Autodesk Fusion 360 part; units mm, degrees
(part 2 of 2)
sketch "Sketch1" plane through (0, 0, 0) normal (0, 0, 1) x (1, 0, 0)
  circle A0 centre (0, 0) radius 2
  circle A1 centre (0, 0) radius 7.85
  dimension "d1" = 4
  dimension "d2" = 15.7
  constraint coincident A0.centre A1.centre
  measures "d1" diameter of A0
  measures "d2" diameter of A1
extrude "Extrude1" add sketch "Sketch1" along normal blind 1 contours A0 | A1
extrude "Extrude2" add sketch "Sketch1" along normal blind 3 contours A0
sketch "Sketch2" plane through (0, 0, 3) normal (0, 0, 1) x (-1, 0, 0)
  circle A0 centre (0, 0) radius 2
  circle A1 centre (0, 0) radius 0.75
  dimension "d7" = 1.5
  constraint concentric A0 A1
  measures "d7" diameter of A1
extrude "Extrude3" cut sketch "Sketch2" against normal blind 7 contours A1
sketch "Sketch3" plane through (0, 0, 3) normal (0, 0, 1) x (-1, 0, 0)
  circle A0 centre (0, 0) radius 0.75
  circle A1 centre (0, 0) radius 2
  circle A2 centre (0, 0) radius 2
  line L0 (0.35, -1.9691) -> (0, -1.3629)
  line L1 (0, -1.3629) -> (-0.35, -1.9691)
  dimension "d10" = 0.7
  dimension "d11" = 0.7
  constraint coincident A0.centre A1.centre
  constraint coincident A1 L0.start
  constraint coincident A2 L1.end
  constraint equal L0 L1
  constraint vertical A0.centre L0.end
  constraint equal A1 A2
  measures "d10" distance of L0.start L0.end
  measures "d11" horizontal distance of L0.start L1.end
extrude "Extrude4" cut sketch "Sketch3" against normal blind 2 contours A1 A2 L0 L1 picked at (0, -1.7853)
pattern_circular "C-Pattern1" count 12 over 360 about axis through (0, 0, 3) along (0, 0, -1) of "Extrude4"
sketch "Sketch4" plane through (0, 0, 1) normal (0, 0, 1) x (-1, 0, 0)
  line L0 (-0.6815, -1.8803) -> (-0.6815, -1.1803)
  line L1 (-0.6815, -1.1803) -> (-1.2877, -1.5303)
  line L2 (-1.5303, -1.2877) -> (-1.1803, -0.6815)
  line L3 (-1.1803, -0.6815) -> (-1.8803, -0.6815)
  line L4 (-1.9691, -0.35) -> (-1.3629, 0)
  line L5 (-1.3629, 0) -> (-1.9691, 0.35)
  line L6 (-1.8803, 0.6815) -> (-1.1803, 0.6815)
  line L7 (-1.1803, 0.6815) -> (-1.5303, 1.2877)
  line L8 (-1.2877, 1.5303) -> (-0.6815, 1.1803)
  line L9 (-0.6815, 1.1803) -> (-0.6815, 1.8803)
  line L10 (-0.35, 1.9691) -> (0, 1.3629)
  line L11 (0, 1.3629) -> (0.35, 1.9691)
  line L12 (0.6815, 1.8803) -> (0.6815, 1.1803)
  line L13 (0.6815, 1.1803) -> (1.2877, 1.5303)
  line L14 (1.5303, 1.2877) -> (1.1803, 0.6815)
  line L15 (1.1803, 0.6815) -> (1.8803, 0.6815)
  line L16 (1.9691, 0.35) -> (1.3629, 0)
  line L17 (1.3629, 0) -> (1.9691, -0.35)
  line L18 (1.8803, -0.6815) -> (1.1803, -0.6815)
  line L19 (1.1803, -0.6815) -> (1.5303, -1.2877)
  line L20 (1.2877, -1.5303) -> (0.6815, -1.1803)
  line L21 (0.6815, -1.1803) -> (0.6815, -1.8803)
  line L22 (0.35, -1.9691) -> (0, -1.3629)
  line L23 (0, -1.3629) -> (-0.35, -1.9691)
  circle A0 centre (0, 0) radius 7.85
  circle A1 centre (0, 0) radius 7.85
  line L24 (0.35, -7.8422) -> (0, -7.236)
  line L25 (0, -7.236) -> (-0.35, -7.8422)
  arc A2 (-0.6815, -1.8803) -> (-0.35, -1.9691) centre (0, 0) ccw
  arc A3 (-1.5303, -1.2877) -> (-1.2877, -1.5303) centre (0, 0) ccw
  arc A4 (-1.9691, -0.35) -> (-1.8803, -0.6815) centre (0, 0) ccw
  arc A5 (-1.8803, 0.6815) -> (-1.9691, 0.35) centre (0, 0) ccw
  arc A6 (-1.2877, 1.5303) -> (-1.5303, 1.2877) centre (0, 0) ccw
  arc A7 (-0.35, 1.9691) -> (-0.6815, 1.8803) centre (0, 0) ccw
  arc A8 (0.6815, 1.8803) -> (0.35, 1.9691) centre (0, 0) ccw
  arc A9 (1.5303, 1.2877) -> (1.2877, 1.5303) centre (0, 0) ccw
  arc A10 (1.9691, 0.35) -> (1.8803, 0.6815) centre (0, 0) ccw
  arc A11 (1.8803, -0.6815) -> (1.9691, -0.35) centre (0, 0) ccw
  arc A12 (1.2877, -1.5303) -> (1.5303, -1.2877) centre (0, 0) ccw
  arc A13 (0.35, -1.9691) -> (0.6815, -1.8803) centre (0, 0) ccw
  dimension "d16" = 0.7
  dimension "d17" = 0.7
  constraint coincident A0.centre A1.centre
  constraint coincident A1 L24.start
  constraint coincident A1 L25.end
  constraint equal L24 L25
  constraint vertical A0.centre L24.end
  constraint equal A0 A1
  measures "d16" distance of L24.start L24.end
  measures "d17" distance of L24.start L25.end
extrude "Extrude5" cut sketch "Sketch4" against normal blind 1.3 contours A0 A1 L24 L25 picked at (0, -7.6447)
pattern_circular "C-Pattern2" count 50 over 360 about axis through (0, 0, 1.75) along (0, 0, 1) of "Extrude5"

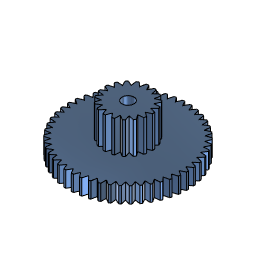
design "MG996R_Gear_3"
Autodesk Fusion 360 part; units mm, degrees
sketch "Sketch1" plane through (0, 0, 0) normal (0, 0, 1) x (1, 0, 0)
  circle A0 centre (0, 0) radius 3
  circle A1 centre (0, 0) radius 7.5
  dimension "d1" = 6
  dimension "d2" = 15
  constraint coincident A0.centre A1.centre
  constraint concentric A0 A1
  measures "d1" diameter of A0
  measures "d2" diameter of A1
extrude "Extrude1" add sketch "Sketch1" along normal blind 6 contours A0
extrude "Extrude2" add sketch "Sketch1" along normal blind 2
sketch "Sketch2" plane through (0, 0, 6) normal (0, 0, 1) x (-1, 0, 0)
  circle A0 centre (0, 0) radius 3
  circle A1 centre (0, 0) radius 0.75
  dimension "d7" = 1.5
  constraint coincident A0.centre A1.centre
  measures "d7" diameter of A1
extrude "Extrude3" cut sketch "Sketch2" against normal blind 14 contours A1
sketch "Sketch3" plane through (0, 0, 2) normal (0, 0, 1) x (-1, 0, 0)
  circle A0 centre (0, 0) radius 3
  circle A1 centre (0, 0) radius 7.5
  circle A2 centre (0, 0) radius 7.5
  line L0 (0.35, -7.4918) -> (0, -6.8856)
  line L1 (0, -6.8856) -> (-0.35, -7.4918)
  dimension "d10" = 0.7
  dimension "d11" = 0.7
  constraint concentric A0 A2
  constraint equal A1 A2
  constraint coincident A2 L0.start
  constraint coincident A2 L1.end
  constraint equal L0 L1
  constraint vertical A0.centre L0.end
  measures "d10" horizontal distance of L0.start L1.end
  measures "d11" distance of L0.start L0.end
extrude "Extrude4" cut sketch "Sketch3" against normal blind 5.5 contours A1 A2 L0 L1 picked at (0, -7.2946)
pattern_circular "C-Pattern1" count 50 over 360 about axis through (0, 0, 6) along (0, 0, -1) of "Extrude4"
sketch "Sketch4" plane through (0, 0, 6) normal (0, 0, 1) x (-1, 0, 0)
  circle A0 centre (0, 0) radius 0.75
  circle A1 centre (0, 0) radius 3
  circle A2 centre (0, 0) radius 3
  line L0 (0.35, -2.9795) -> (0, -2.3733)
  line L1 (0, -2.3733) -> (-0.35, -2.9795)
  dimension "d16" = 0.7
  dimension "d17" = 0.7
  constraint concentric A0 A2
  constraint equal A1 A2
  constraint coincident A1 L0.start
  constraint coincident A2 L1.end
  constraint vertical A0.centre L0.end
  constraint equal L0 L1
  measures "d16" distance of L0.start L0.end
  measures "d17" horizontal distance of L0.start L1.end
extrude "Extrude5" cut sketch "Sketch4" against normal blind 4 contours A1 A2 L0 L1 picked at (0, -2.7896)
pattern_circular "C-Pattern2" count 19 over 360 about axis through (0, 0, 6) along (0, 0, -1) of "Extrude5"

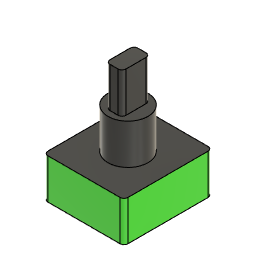
design "MG996R_Pot"
Autodesk Fusion 360 part; units mm, degrees
sketch "Sketch1" plane through (0, 0, 0) normal (0, 0, 1) x (1, 0, 0)
  line L0 (5, 5.5) -> (-5, 5.5)
  line L1 (-5, 5.5) -> (-5, -5.5)
  line L2 (-5, -5.5) -> (5, -5.5)
  line L3 (5, -5.5) -> (5, 5.5)
  line L4 (5, 5.5) -> (-5, -5.5) construction
  line L5 (-5, 5.5) -> (5, -5.5) construction
  dimension "d1" = 10
  dimension "d2" = 11
  constraint horizontal L0
  constraint perpendicular L0 L1
  constraint parallel L0 L2
  constraint parallel L1 L3
  constraint coincident L4 origin
  constraint coincident L5 origin
  measures "d1" distance of L0.start L0.end
  measures "d2" distance of L0.end L1.end
extrude "Extrude1" add sketch "Sketch1" along normal blind 5
sketch "Sketch2" plane through (0, 0, 5) normal (0, 0, 1) x (-1, 0, 0)
  line L0 (-5, 5.5) -> (-5, -5.5)
  line L1 (-5, -5.5) -> (5, -5.5)
  line L2 (5, -5.5) -> (5, 5.5)
  line L3 (5, 5.5) -> (-5, 5.5)
  circle A0 centre (0, 0) radius 2.5
  dimension "d5" = 5
  constraint coincident A0.centre origin
  measures "d5" diameter of A0
extrude "Extrude2" add sketch "Sketch2" along normal blind 10 contours A0
sketch "Sketch3" plane through (0, 0, 15) normal (0, 0, 1) x (-1, 0, 0)
  circle A0 centre (0, 0) radius 2.5
  line L0 (-1, -1.75) -> (1, -1.75)
  line L1 (1, -1.75) -> (1, 1.75)
  line L2 (1, 1.75) -> (-1, 1.75)
  line L3 (-1, 1.75) -> (-1, -1.75)
  line L4 (-1, -1.75) -> (1, 1.75) construction
  line L5 (1, -1.75) -> (-1, 1.75) construction
  dimension "d8" = 2
  dimension "d9" = 3.5
  constraint horizontal L0
  constraint perpendicular L0 L1
  constraint parallel L0 L2
  constraint parallel L1 L3
  constraint coincident L4 A0.centre
  constraint coincident L5 A0.centre
  constraint coincident A0.centre origin
  measures "d8" distance of L1 L3
  measures "d9" distance of L0.end L1.end
extrude "Extrude3" cut sketch "Sketch3" against normal blind 5
fillet "Fillet1" radius 0.5 4 edges at (-1, -1.75, 12.5) (1, -1.75, 12.5) (-1, 1.75, 12.5) (1, 1.75, 12.5)
fillet "Fillet2" radius 0.5 4 edges at (-5, 5.5, 2.5) (5, 5.5, 2.5) (-5, -5.5, 2.5) (5, -5.5, 2.5)

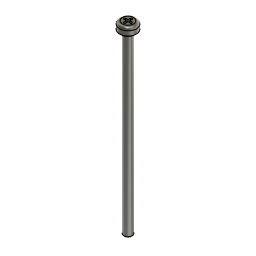
design "MG996R_Screw"
Autodesk Fusion 360 part; units mm, degrees
sketch "Sketch1" plane through (0, 0, 0) normal (0, 0, 1) x (1, 0, 0)
  circle A0 centre (0, 0) radius 0.75
  dimension "d1" = 1.5
  constraint coincident A0.centre origin
  measures "d1" diameter of A0
extrude "Extrude1" add sketch "Sketch1" along normal blind 33
sketch "Sketch2" plane through (0, 0, 33) normal (0, 0, 1) x (-1, 0, 0)
  circle A0 centre (0, 0) radius 0.75
  circle A1 centre (0, 0) radius 1.5
  dimension "d4" = 3
  constraint concentric A0 A1
  measures "d4" diameter of A1
extrude "Extrude2" add sketch "Sketch2" against normal blind 1.5
fillet "Fillet1" radius 0.5 1 edges at (1.3985, 0.5424, 33)
fillet "Fillet2" radius 0.2 1 edges at (1.3985, -0.5424, 31.5)
sketch "Sketch3" plane through (0, 0, 33) normal (0, 0, 1) x (-1, 0, 0)
  circle A0 centre (0, 0) radius 1
  line L0 (0.6, 0.15) -> (-0.6, 0.15)
  arc A1 (-0.6, 0.15) -> (-0.6, -0.15) centre (-0.6, 0) ccw
  line L1 (-0.6, -0.15) -> (0.6, -0.15)
  arc A2 (0.6, -0.15) -> (0.6, 0.15) centre (0.6, 0) ccw
  line L2 (0.6, 0) -> (-0.6, 0) construction
  line L3 (-0.15, 0.6) -> (-0.15, -0.6)
  arc A3 (-0.15, -0.6) -> (0.15, -0.6) centre (0, -0.6) ccw
  line L4 (0.15, -0.6) -> (0.15, 0.6)
  arc A4 (0.15, 0.6) -> (-0.15, 0.6) centre (0, 0.6) ccw
  line L5 (0, 0.6) -> (0, -0.6) construction
  dimension "d11" = 0.3
  dimension "d12" = 1.2
  dimension "d13" = 0.3
  dimension "d14" = 1.2
  constraint tangent L0 A1
  constraint tangent A1 L1
  constraint parallel L0 L1
  constraint tangent L1 A2
  constraint tangent L0 A2
  constraint horizontal L2
  constraint coincident A0.centre origin
  constraint midpoint L2 A0.centre
  constraint tangent L3 A3
  constraint tangent A3 L4
  constraint parallel L3 L4
  constraint tangent L4 A4
  constraint tangent L3 A4
  constraint perpendicular L1 L5
  constraint midpoint L5 A0.centre
  measures "d11" distance of L0 L1
  measures "d12" distance of A1.end L1.end
  measures "d13" distance of L3 L4
  measures "d14" distance of A4.centre A3.centre
extrude "Extrude3" cut sketch "Sketch3" against normal blind 1.2 contours L0 L1 A2 L4 | L0 L1 L3 L4 | L0 L3 L4 A4 | L0 A1 L1 L3 | L1 L3 A3 L4
fillet "Fillet3" radius 0.3 1 edges at (-0.6992, -0.2712, 0)
